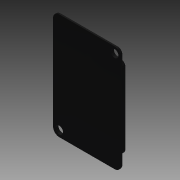
# Autodesk Inventor part: IO-Shield-Sideplate01
Saved by Autodesk Inventor 2013 (Build 170138000, 138)
## iProperties
Created: 2015-02-10
Part Number: IO-Shield-Sideplate01
Material: Generic
Document SubType Name: Modeling
Designer: spichelh
Density: 1 g/cm^3
Author: spichelh
Autodesk Inventor part; units mm, degrees
ref_plane "YZ Plane" through (0, 0, 0) normal (1, 0, 0) x (0, 1, 0)
ref_plane "XZ Plane" through (0, 0, 0) normal (0, 1, 0) x (-1, 0, 0)
ref_plane "XY Plane" through (0, 0, 0) normal (0, 0, 1) x (1, 0, 0)
sketch "Sketch1" plane through (0, 0, 0) normal (0, 0, 1) x (1, 0, 0)
  line L0 (0, -24.5) -> (-18, -24.5)
  line L1 (-20, -22.5) -> (-20, 0)
  line L2 (-18, 2) -> (0, 2)
  line L3 (2, 0) -> (2, -22.5)
  arc A0 (-18, 2) -> (-20, 0) centre (-18, 0) ccw
  arc A1 (2, 0) -> (0, 2) centre (0, 0) ccw
  arc A2 (0, -24.5) -> (2, -22.5) centre (0, -22.5) ccw
  arc A3 (-20, -22.5) -> (-18, -24.5) centre (-18, -22.5) ccw
  dimension "d0" = 2
  dimension "d1" = 22
  dimension "d2" = 26.5
  constraints: 8 end point, 8 point on circle, 8 tangent, 4 centre point, 3 equal radius, 2 parallel, 1 coincident, 1 horizontal, 1 perpendicular
  measures "d0" radius of A0
  measures "d1" distance between parallel lines of L1 L3
  measures "d2" distance between parallel lines of L2 L0
extrude "Extrusion1" add sketch "Sketch1" along normal blind 1
sketch "Sketch2" plane through (0, 0, 1) normal (0, 0, 1) x (1, 0, 0)
  line L0 (-20, 0) -> (-20, -22.5) projected
  line L1 (-18, -24.5) -> (0, -24.5) projected
  line L2 (2, -22.5) -> (2, 0) projected
  line L3 (0, 2) -> (-18, 2) projected
  line L4 (-18, 6) -> (0, 6)
  line L5 (2, 4) -> (2, -26.5)
  line L6 (0, -28.5) -> (-18, -28.5)
  line L7 (-20, -26.5) -> (-20, 4)
  arc A0 (0, -28.5) -> (2, -26.5) centre (0, -26.5) ccw
  arc A1 (-20, -26.5) -> (-18, -28.5) centre (-18, -26.5) ccw
  arc A2 (-18, 6) -> (-20, 4) centre (-18, 4) ccw
  arc A3 (2, 4) -> (0, 6) centre (0, 4) ccw
  circle A4 centre (-18, -26.5) radius 1.25
  circle A5 centre (0, 4) radius 1.25
  point P0 (0, 0)
  dimension "d5" = 2
  dimension "d6" = 4
  dimension "d7" = 4
  dimension "d8" = 2.5
  dimension "d9" = 2.5
  dimension "d18" = 34.5
  dimension "d19" = 26.5
  dimension "d20" = 22
  constraints: 8 end point, 8 point on circle, 8 tangent, 6 centre point, 3 equal radius, 2 coincident, 2 collinear, 2 parallel, 1 horizontal, 1 perpendicular
  measures "d5" radius of A0
  measures "d6" distance between parallel lines of L4 L3
  measures "d7" distance between parallel lines of L6 L1
  measures "d8" diameter of A4
  measures "d9" diameter of A5
  measures "d18" distance between parallel lines of L6 L4
  measures "d19" distance between parallel lines of L3 L1
  measures "d20" distance between parallel lines of L2 L7
extrude "Extrusion2" add sketch "Sketch2" along normal blind 1
chamfer "Chamfer1" distance 0.5 angle 45 8 edges at (-19.4142, 1.4142, 0) (-20, -11.25, 0) (-19.4142, -23.9142, 0) (-9, -24.5, 0) (1.4142, -23.9142, 0) (2, -11.25, 0) (1.4142, 1.4142, 0) (-9, 2, 0)
chamfer "Chamfer2" distance 0.5 angle 45 10 edges at (-20, -24.5, 1) (-19.4142, -27.9142, 1) (-9, -28.5, 1) (1.4142, -27.9142, 1) (2, -24.5, 1) (-20, 2, 1) (-19.4142, 5.4142, 1) (-9, 6, 1) (1.4142, 5.4142, 1) (2, 2, 1)
body "Solid1"
